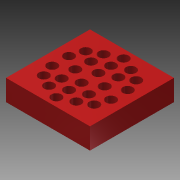
# Autodesk Inventor part: FanTemplate40mm
Saved by Autodesk Inventor 2015 SP1 (Build 190203100, 203)
## iProperties
Created: 2015-04-15
Part Number: FanTemplate40mm
Material: Generic
Document SubType Name: Modeling
Designer: Jack
Density: 1 g/cm^3
Appearance: Light Red
Author: Jack
Autodesk Inventor part; units mm, degrees
ref_plane "YZ Plane" through (0, 0, 0) normal (1, 0, 0) x (0, 1, 0)
ref_plane "XZ Plane" through (0, 0, 0) normal (0, 1, 0) x (-1, 0, 0)
sketch "Sketch1" plane through (0, 0, 0) normal (0, 0, 1) x (1, 0, 0)
  line L0 (-20, -20) -> (20, -20)
  line L1 (20, -20) -> (20, 20)
  line L2 (20, 20) -> (-20, 20)
  line L3 (-20, 20) -> (-20, -20)
  line L4 (-20, -20) -> (20, 20) construction
  line L5 (20, -20) -> (-20, 20) construction
  point P0 (0, 0)
  dimension "d0" = 40
  dimension "d1" = 40
  constraints: 12 end point, 2 midpoint, 2 parallel, 1 horizontal, 1 perpendicular
  measures "d0" distance of L2.end L1.end
  measures "d1" distance of L1.end L0.end
extrude "Extrusion1" add sketch "Sketch1" along normal blind 10
sketch "Sketch2" plane through (0, 0, 10) normal (0, 0, 1) x (1, 0, 0)
  circle A0 centre (0, 0) radius 19
  line L0 (-10.247, 16) -> (10.247, 16)
  line L1 (-13.8564, 13) -> (13.8564, 13)
  line L2 (-16.1555, 10) -> (16.1555, 10)
  line L3 (-17.6635, 7) -> (17.6635, 7)
  line L4 (-18.5742, 4) -> (18.5742, 4)
  circle A1 centre (0, 16) radius 2.38
  circle A2 centre (-6.5, 13) radius 2.38
  circle A3 centre (6.5, 13) radius 2.38
  circle A4 centre (-12, 10) radius 2.38
  circle A5 centre (0, 10) radius 2.38
  circle A6 centre (12, 10) radius 2.38
  circle A7 centre (-6.5, 7) radius 2.38
  circle A8 centre (6.5, 7) radius 2.38
  circle A9 centre (-14, 4) radius 2.38
  circle A10 centre (0, 4) radius 2.38
  circle A11 centre (14, 4) radius 2.38
  circle A12 centre (-7, 0) radius 2.38
  circle A13 centre (7, 0) radius 2.38
  dimension "d4" = 38
  dimension "d5" = 4.76
  dimension "d6" = 4.76
  dimension "d7" = 4.76
  dimension "d8" = 3
  dimension "d9" = 3
  dimension "d10" = 16
  dimension "d11" = 6.5
  dimension "d12" = 6.5
  dimension "d13" = 12
  dimension "d14" = 12
  dimension "d15" = 3
  dimension "d16" = 3
  dimension "d17" = 14
  dimension "d18" = 14
  dimension "d19" = 7
  dimension "d20" = 7
  constraints: 13 centre point, 10 end point, 10 equal radius, 8 point on line, 3 midpoint, 3 parallel, 3 vertical alignment, 2 horizontal, 2 horizontal alignment, 1 coincident, 12 other
  measures "d5" diameter of A2
  measures "d6" diameter of A1
  measures "d7" diameter of A3
  measures "d8" distance between parallel lines of L0 L1
  measures "d9" distance between parallel lines of L1 L2
  measures "d10" distance from line of point (0, 0) L0
  measures "d11" horizontal distance of A1.centre A2.centre
  measures "d12" horizontal distance of A3.centre A1.centre
  measures "d13" distance of A6.centre A5.centre
  measures "d14" distance of A5.centre A4.centre
  measures "d15" distance between parallel lines of L2 L3
  measures "d16" distance between parallel lines of L3 L4
  measures "d17" distance of A10.centre A9.centre
  measures "d18" distance of A11.centre A10.centre
  measures "d19" horizontal distance of A10.centre A12.centre
  measures "d20" horizontal distance of A10.centre A13.centre
extrude "Extrusion2" cut sketch "Sketch2" against normal up to next contours A11 L4 | L4 A11 | A9 L4 | L4 A9 | A8 L3 | L3 A8 | A7 L3 | L3 A7 | A6 L2 | L2 A6 | A10 L4 | L4 A10 | A4 L2 | L2 A4 | A3 L1 | L1 A3 | A2 L1 | L1 A2 | A1 L0 | L0 A1 | A5 L2 | L2 A5 | A12 | A13
ref_plane "Work Plane1" through (-20, 0, 0) normal (0, 1, 0) x (1, 0, 0)
mirror "Mirror1" about plane through (-20, 0, 0) normal (0, 1, 0) of "Extrusion2"
body "Solid1"
